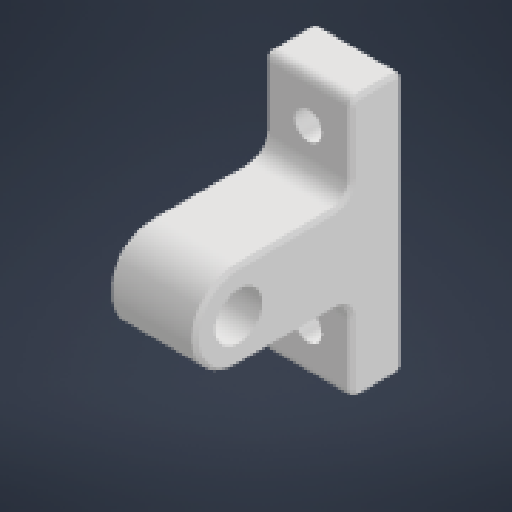
# Autodesk Inventor part: SoporteEjeMotor
Saved by Autodesk Inventor 2026.2 (Build 302298010, 298A)
## iProperties
Created: 2026-04-29
Part Number: SoporteEjeMotor
Material: Genérico
Document SubType Name: Modeling
Designer: Jose Carlos
Density: 1 g/cm^3
Appearance: Valor por defecto
Author: Jose Carlos
Autodesk Inventor part; units mm, degrees
ref_plane "YZ Plane" through (0, 0, 0) normal (1, 0, 0) x (0, 1, 0)
ref_plane "XZ Plane" through (0, 0, 0) normal (0, 1, 0) x (-1, 0, 0)
ref_plane "Plano de trabajo1" through (-7.3035, 18.7537, -25.5454) normal (-1, 0, 0) x (0, 1, 0)
sketch "Boceto1" plane through (-7.3035, 18.7537, -25.5454) normal (-1, 0, 0) x (0, 1, 0)
  line L0 (40.0076, 19) -> (-60.0081, 19) construction
  line L1 (15, 19) -> (-15, 19)
  line L2 (-15, 19) -> (-15, 13)
  line L3 (-15, 13) -> (15, 13)
  line L4 (15, 13) -> (15, 19)
  line L5 (-5, 19) -> (5, 19)
  line L6 (5, 19) -> (5, -5)
  line L7 (5, -5) -> (-5, -5)
  line L8 (-5, -5) -> (-5, 19)
  arc A0 (-1.0724, -0.9) -> (-0.9, -1.0724) centre (0, 0) ccw construction
  circle A1 centre (0, 0) radius 2.7
  point P0 (-18.7537, -25.5454)
  point P1 (0, 19)
  point P2 (0, -5)
  point P3 (-5, 13)
  point P4 (5, 13)
  dimension "d0" = 6
  dimension "d1" = 30
  dimension "d2" = 5.4
  dimension "d3" = 0
  dimension "d4" = 0
  dimension "d5" = 10
  dimension "d6" = 5
  constraints: 16 end point, 4 parallel, 2 horizontal, 2 midpoint, 2 perpendicular, 2 point on line, 1 centre point, 1 coincident
  measures "d0" distance of L3.end L1.start
  measures "d1" distance of L2.end L3.end
  measures "d2" diameter of A1
  measures "d3" horizontal distance of A0.centre point (0, 19)
  measures "d4" horizontal distance of A0.centre point (0, -5)
  measures "d5" distance of L6.end L7.end
  measures "d6" distance from line of A0.centre L7
extrude "Extrusión1" add sketch "Boceto1" against normal blind 10
sketch "Boceto2" plane through (-7.3035, 23.7537, -38.5454) normal (0, 0, 1) x (1, 0, 0)
  line L0 (0, 0) -> (10, 0) construction
  line L1 (0, 0) -> (0, 10) construction
  line L2 (0, -20) -> (0, -10) construction
  line L3 (0, -10) -> (10, -10) construction
  point P0 (7.3035, -23.7537)
  point P1 (5, 5)
  point P2 (5, -15)
  point P3 (5, 0)
  point P4 (5, -10)
  dimension "d9" = 5
  dimension "d10" = 5
  dimension "d11" = 5
  dimension "d12" = 5
  constraints: 2 midpoint
  measures "d9" distance of point (5, 0) point (5, 5)
  measures "d10" distance from line of L1 point (5, 5)
  measures "d11" distance from line of L2 point (5, -15)
  measures "d12" distance of point (5, -10) point (5, -15)
hole "Agujero1" at (-2.3035, 28.7537, -38.5454) at (-2.3035, 8.7537, -38.5454) direction (0, 0, -1) diameter 3.2 end through all
fillet "Empalme1" radius 5 2 edges at (-2.3035, 23.7537, -20.5454) (-2.3035, 13.7537, -20.5454)
fillet "Empalme2" radius 1 4 edges at (-2.3035, 33.7537, -38.5454) (-2.3035, 3.7537, -38.5454) (-2.3035, 33.7537, -44.5454) (-2.3035, 3.7537, -44.5454)
fillet "Empalme3" radius 2 2 edges at (-2.3035, 23.7537, -38.5454) (-2.3035, 13.7537, -38.5454)
chamfer "Chaflán1" distance 0.4 angle 45 24 edges at (-7.3035, 29.2537, -38.5454) (-7.3035, 33.4608, -38.8383) (-7.3035, 33.7537, -41.5454) (-7.3035, 33.4608, -44.2525) (-7.3035, 18.7537, -44.5454) (-7.3035, 4.0466, -44.2525) (-7.3035, 3.7537, -41.5454) (-7.3035, 4.0466, -38.8383) (-7.3035, 8.2537, -38.5454) (-7.3035, 13.7537, -31.0451) (-7.3035, 22.2894, -22.0097) (-7.3035, 23.7537, -31.0451) (2.6965, 29.2537, -38.5454) (2.6965, 23.7537, -31.0451) (2.6965, 22.2894, -22.0097) (2.6965, 13.7537, -31.0451) (2.6965, 8.2537, -38.5454) (2.6965, 4.0466, -38.8383) (2.6965, 3.7537, -41.5454) (2.6965, 4.0466, -44.2525) (2.6965, 18.7537, -44.5454) (2.6965, 33.4608, -44.2525) (2.6965, 33.7537, -41.5454) (2.6965, 33.4608, -38.8383)
